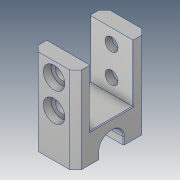
# Autodesk Inventor part: 200-50-WHEEL-CONNECTOR-30MM-01
Saved by Autodesk Inventor 2018.2 (Build 222227000, 227)
## iProperties
Manager: feesmrt
Company: FRANC0R
Created: 2017-12-05
Part Number: 200-50-WHEEL-CONNECTOR-30MM-01
Material: Aluminium 6061
Document SubType Name: Modeling
Designer: feesmrt
Density: 2.7 g/cm^3
Appearance: Aluminium - flach
Project: Rescue Robot
Cost Center: -
Engineer: feesmrt
Authority: feesmrt
Description: Wheel Connector 30mm Part 1
Stock Number: 200-50-WHEEL-CONNECTOR-30MM-01
Author: feesmrt
Subject: Rescue Robot
Title: Wheel Connector 30mm Part 1
Revision Number: 1
Autodesk Inventor part; units mm, degrees
note: some values were not read from the file. Chosen so that the rebuilt part matches the saved one: direction of "DIN7984_M8_Boh".
ref_plane "YZ Plane" through (0, 0, 0) normal (1, 0, 0) x (0, 1, 0)
ref_plane "XZ Plane" through (0, 0, 0) normal (0, 1, 0) x (-1, 0, 0)
ref_plane "XY Plane" through (0, 0, 0) normal (0, 0, 1) x (1, 0, 0)
sketch "Skizze1" plane through (0, 0, 0) normal (1, 0, 0) x (0, 1, 0)
  line L0 (-35, 0) -> (35, 0) construction
  line L1 (0, 42) -> (0, -42) construction
  line L2 (-25, -30) -> (25, -30)
  line L3 (25, -30) -> (25, 30)
  line L4 (25, 30) -> (-25, 30)
  line L5 (-25, 30) -> (-25, -30)
  line L6 (-25, -30) -> (25, 30) construction
  line L7 (25, -30) -> (-25, 30) construction
  point P0 (0, 0)
  dimension "d0" = 50
  dimension "d1" = 60
  constraints: 12 end point, 2 midpoint, 2 parallel, 1 horizontal, 1 perpendicular
  measures "d0" distance of L3.end L4.end
  measures "d1" distance of L2.end L3.end
extrude "Grundkörper" add sketch "Skizze1" along normal mid plane 30
sketch "Skizze2" plane through (15, 0, 0) normal (1, 0, 0) x (0, 0, -1)
  line L0 (-30, 25) -> (-30, -25) construction
  line L1 (0, -35) -> (0, 35) construction
  line L2 (-42, 0) -> (42, 0) construction
  line L3 (-30, -15) -> (10, -15)
  line L4 (10, -15) -> (10, 15)
  line L5 (10, 15) -> (-30, 15)
  line L6 (-30, 15) -> (-30, -15)
  line L7 (30, -25) -> (30, 25) construction
  line L8 (30, -8.4) -> (25, -8.4)
  line L9 (17, -0.4) -> (17, 0.4)
  line L10 (25, 8.4) -> (30, 8.4)
  line L11 (30, -8.4) -> (30, 8.4)
  arc A0 (17, -0.4) -> (25, -8.4) centre (25, -0.4) ccw
  arc A1 (25, 8.4) -> (17, 0.4) centre (25, 0.4) ccw
  point P0 (0, 0)
  dimension "d4" = 40
  dimension "d5" = 30
  dimension "d14" = 13
  dimension "d15" = 16.8
  dimension "d16" = 8
  constraints: 16 end point, 4 perpendicular, 4 point on circle, 4 tangent, 3 point on line, 2 centre point, 2 horizontal, 2 parallel, 1 equal radius, 2 other
  measures "d4" distance of L3.start L3.end
  measures "d5" distance between parallel lines of L5 L3
  measures "d14" distance between parallel lines of L7 L9
  measures "d15" distance between parallel lines of L8 L10
  measures "d16" radius of A0
extrude "Ausschnitt" cut sketch "Skizze2" against normal through all
sketch "Skizze4" plane through (-15, -25, -30) normal (0, -1, 0) x (1, 0, 0)
  line L0 (30, 20) -> (0, 20) construction
  line L1 (30, 60) -> (0, 60) construction
  line L2 (15, 72) -> (15, -12) projected
  line L3 (0, 40) -> (30, 40) construction
  line L4 (0, 0) -> (0, 60) construction
  line L5 (30, 60) -> (30, 0) construction
  point P0 (15, 30)
  point P1 (15, 50)
  point P2 (15, 30)
  dimension "d19" = 40
  dimension "d20" = 20
  dimension "d21" = 20
  constraints: 3 point on line, 2 end point, 1 horizontal, 1 midpoint, 1 symmetric about line
  measures "d19" distance between parallel lines of L0 L1
  measures "d20" distance between parallel lines of L1 L3
  measures "d21" distance of point (15, 30) point (15, 50)
hole "DIN7984_M8_Boh" at (0, -25, 20) at (0, -25, 0) direction (0, 1, 0) diameter 9 end up to surface counterbore diameter 15 counterbore depth 5.4
mirror "Spiegeln_DIN7984_M8_Boh" about plane through (0, 0, 0) normal (0, 1, 0) of "DIN7984_M8_Boh"
sketch "Skizze5" plane through (15, -25, -30) normal (0, 0, -1) x (-1, 0, 0)
  line L0 (0, 0) -> (30, 0) construction
  line L1 (30, 16.6) -> (0, 16.6) construction
  line L2 (30, 50) -> (0, 50) construction
  line L3 (0, 33.4) -> (30, 33.4) construction
  line L4 (15, -10) -> (15, 60) construction
  line L5 (-6, 25) -> (36, 25) construction
  line L6 (15, 16.6) -> (15, 0) construction
  point P0 (15, 25)
  point P1 (15, 8.3)
  point P2 (15, 41.7)
  dimension "d29" = 33.4
  constraints: 3 midpoint, 2 end point, 2 point on line, 1 symmetric about line
  measures "d29" distance of point (15, 41.7) point (15, 8.3)
hole "M5x10" at (0, -16.7, -30) at (0, 16.7, -30) direction (0, 0, 1) diameter 4.134 depth 14.2 tip angle 118 countersink diameter 5 countersink angle 90 thread size "M5x0.8" class "6H" standard "ISO Metric profile"
sketch "Skizze" plane through (15, -25, -30) normal (0, 0, -1) x (-1, 0, 0)
  circle A0 centre (15, 8.3) radius 2.5 projected
  line L0 (30, 16.6) -> (0, 16.6) projected
  line L1 (0, 0) -> (0, 16.6) projected
  line L2 (0, 0) -> (30, 0) projected
  line L3 (30, 16.6) -> (30, 0) projected
  circle A1 centre (15, 41.7) radius 2.5 projected
  line L4 (0, 33.4) -> (30, 33.4) projected
  line L5 (30, 50) -> (30, 33.4) projected
  line L6 (30, 50) -> (0, 50) projected
  line L7 (0, 33.4) -> (0, 50) projected
  line L8 (0, 16.6) -> (0, 24.6) projected
  line L9 (0, 24.6) -> (0, 25.4) projected
  line L10 (0, 25.4) -> (0, 33.4) projected
  line L11 (30, 33.4) -> (30, 25.4) projected
  line L12 (30, 25.4) -> (30, 24.6) projected
  line L13 (30, 24.6) -> (30, 16.6) projected
  point P0 (15, 25)
chamfer "Fase_Allgemein" distance 4 angle 45 4 edges at (15, -25, 0) (-15, -25, 0) (15, 25, 0) (-15, 25, 0)
chamfer "Fase" distance 0.5 angle 45 15 edges at (15, -6.0569, -19.3431) (15, 0, -17) (15, 6.0569, -19.3431) (15, 8.4, -27.5) (15, -8.4, -27.5) (-15, 6.0569, -19.3431) (-15, 0, -17) (-15, -6.0569, -19.3431) (-15, -8.4, -27.5) (-15, 8.4, -27.5) (-15, 0, -10) (-15, 15, 10) (15, -15, 10) (15, 0, -10) (15, 15, 10)
equation "\"d20\" = 0.5 * d19"
equation "\"d21\" = 0.5 * d19"
